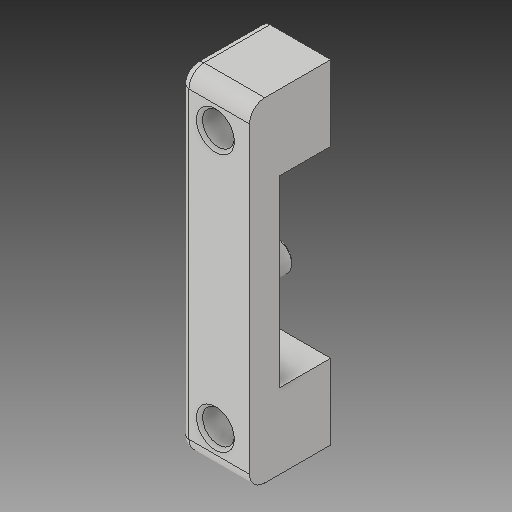
# Autodesk Inventor part: servo_cap
Saved by Autodesk Inventor 2019 (Build 230136000, 136)
## iProperties
Created: 2021-10-06
Part Number: servo_cap
Material: Generic
Document SubType Name: Modeling
Designer: Pokick
Density: 1 g/cm^3
Appearance: Default
Author: Pokick
Autodesk Inventor part; units mm, degrees
ref_plane "YZ Plane" through (0, 0, 0) normal (1, 0, 0) x (0, 1, 0)
ref_plane "XZ Plane" through (0, 0, 0) normal (0, 1, 0) x (-1, 0, 0)
ref_plane "XY Plane" through (0, 0, 0) normal (0, 0, 1) x (1, 0, 0)
sketch "Sketch1" plane through (0, 0, 0) normal (0, 0, 1) x (1, 0, 0)
  line L0 (-2.25, -11) -> (2.25, -11)
  line L1 (2.25, -11) -> (2.25, 11)
  line L2 (2.25, 11) -> (-2.25, 11)
  line L3 (-2.25, 11) -> (-2.25, -11)
  line L4 (-2.25, -11) -> (2.25, 11) construction
  line L5 (2.25, -11) -> (-2.25, 11) construction
  line L6 (-2.25, 6.05) -> (2.25, 6.05)
  line L7 (2.25, 6.05) -> (2.25, -6.05)
  line L8 (2.25, -6.05) -> (-2.25, -6.05)
  line L9 (-2.25, -6.05) -> (-2.25, 6.05)
  line L10 (-2.25, 6.05) -> (2.25, -6.05) construction
  line L11 (2.25, 6.05) -> (-2.25, -6.05) construction
  point P0 (0, 0)
  dimension "d0" = 4.5
  dimension "d1" = 22
  dimension "d2" = 4.5
  dimension "d3" = 12.1
  constraints: 24 end point, 4 midpoint, 4 parallel, 2 horizontal, 2 perpendicular
  measures "d0" distance of L2.end L1.end
  measures "d1" distance of L1.end L0.end
  measures "d2" distance of L7.end L8.end
  measures "d3" distance of L6.end L7.end
extrude "Extrusion1" add sketch "Sketch1" along normal blind 3.35 contours L3 L8 L1 L0 | L3 L2 L1 L6
sketch "Sketch2" plane through (0, 0, 3.35) normal (0, 0, 1) x (1, 0, 0)
  line L0 (2.25, 6.05) -> (2.25, 11) projected
  line L1 (-2.25, -11) -> (2.25, -11)
  line L2 (2.25, -11) -> (2.25, 11)
  line L3 (2.25, 11) -> (-2.25, 11)
  line L4 (-2.25, 11) -> (-2.25, -11)
  line L5 (-2.25, -11) -> (2.25, 11) construction
  line L6 (2.25, -11) -> (-2.25, 11) construction
  point P0 (0, 0)
  constraints: 12 end point, 2 midpoint, 2 parallel, 1 horizontal, 1 perpendicular
extrude "Extrusion2" add sketch "Sketch2" along normal blind 2
sketch "Sketch3" plane through (0, 0, 3.35) normal (0, 0, -1) x (-1, 0, 0)
  line L0 (0, 0) -> (-0.65, 0) construction
  circle A0 centre (-0.65, 0) radius 0.975
  dimension "d8" = 0.65
  dimension "d9" = 1.95
  constraints: 2 end point, 1 centre point, 1 coincident, 1 horizontal
  measures "d8" distance of L0.start L0.end
  measures "d9" diameter of A0
extrude "Extrusion3" add sketch "Sketch3" along normal blind 1.5
fillet "Fillet1" radius 0.1 2 edges at (1.625, 0, 1.85) (1.625, 0, 3.35)
fillet "Fillet2" radius 1 2 edges at (0, -11, 5.35) (0, 11, 5.35)
sketch "Sketch4" plane through (0, 0, 0) normal (0, 0, -1) x (-1, 0, 0)
  line L0 (-2.25, 11) -> (2.25, 11) construction
  line L1 (-2.25, -11) -> (2.25, -11) construction
  line L2 (2.25, -11) -> (2.25, 11) construction
  line L3 (2.25, 11) -> (-2.25, 11) construction
  line L4 (-2.25, 11) -> (-2.25, -11) construction
  line L5 (-2.25, -11) -> (2.25, 11) construction
  line L6 (2.25, -11) -> (-2.25, 11) construction
  line L7 (0, 0) -> (0, 8.5) construction
  line L8 (2.25, 10) -> (-2.25, 10) projected
  circle A0 centre (0, 8.5) radius 1.05
  dimension "d14" = 8.5
  dimension "d15" = 2.1
  constraints: 14 end point, 2 midpoint, 2 parallel, 2 perpendicular, 1 centre point, 1 coincident, 1 horizontal
  measures "d14" distance of L7.start L7.end
  measures "d15" diameter of A0
extrude "Extrusion4" cut sketch "Sketch4" against normal blind 6
chamfer "Chamfer1" distance 0.2 angle 45 1 edges at (1.05, 8.5, 5.35)
pattern_linear "Rectangular Pattern1" count 2 spacing 17 along (0, -1, 0) of "Extrusion4", "Chamfer1"
fillet "Fillet3" radius 0.5 8 edges at (-2.25, -10.7071, 5.0571) (-2.25, -11, 2.175) (-2.25, 10.7071, 5.0571) (-2.25, 11, 2.175) (-2.25, 0, 5.35) (-2.25, 6.05, 1.675) (-2.25, 0, 3.35) (-2.25, -6.05, 1.675)
body "Solid1"
